Autodesk Inventor part; units mm, degrees
(part 2 of 3)
  line L905 (15.1918, 12.9829) -> (15.4759, 13.083)
  line L906 (15.4759, 13.083) -> (15.7953, 13.1808)
  line L907 (15.7953, 13.1808) -> (16.149, 13.2732)
  line L908 (16.149, 13.2732) -> (16.5404, 13.3581)
  line L909 (16.5404, 13.3581) -> (16.9661, 13.4319)
  line L910 (16.9661, 13.4319) -> (17.3813, 13.4867)
  arc A20 (18.1977, 12.3629) -> (17.3813, 13.4867) centre (0, 0) ccw
  line L911 (18.1977, 12.3629) -> (18.0173, 11.985)
  line L912 (18.0173, 11.985) -> (17.8155, 11.603)
  line L913 (17.8155, 11.603) -> (17.6139, 11.257)
  line L914 (17.6139, 11.257) -> (17.4167, 10.9491)
  line L915 (17.4167, 10.9491) -> (17.225, 10.6756)
  line L916 (17.225, 10.6756) -> (17.042, 10.4364)
  line L917 (17.042, 10.4364) -> (16.8707, 10.231)
  line L918 (16.8707, 10.231) -> (16.7119, 10.0559)
  line L919 (16.7119, 10.0559) -> (16.5707, 9.9128)
  line L920 (16.5707, 9.9128) -> (16.3443, 9.7094)
  line L921 (16.3443, 9.7094) -> (16.2048, 9.6033)
  line L922 (16.2048, 9.6033) -> (16.0637, 9.5056)
  line L923 (16.0637, 9.5056) -> (15.8979, 9.3692)
  line L924 (15.8979, 9.3692) -> (15.7712, 9.237)
  line L925 (15.7712, 9.237) -> (15.7224, 9.1734)
  line L926 (15.7224, 9.1734) -> (15.6831, 9.112)
  line L927 (15.6831, 9.112) -> (15.6531, 9.0532)
  line L928 (15.6531, 9.0532) -> (15.6325, 8.9973)
  line L929 (15.6325, 8.9973) -> (15.621, 8.9446)
  line L930 (15.621, 8.9446) -> (15.6184, 8.8956)
  line L931 (15.6184, 8.8956) -> (15.6247, 8.8505)
  line L932 (15.6247, 8.8505) -> (15.6447, 8.8003)
  line L933 (15.6447, 8.8003) -> (15.7975, 8.5231)
  line L934 (15.7975, 8.5231) -> (15.9936, 8.1491)
  line L935 (15.9936, 8.1491) -> (16.1809, 7.7707)
  line L936 (16.1809, 7.7707) -> (16.3153, 7.4841)
  line L937 (16.3153, 7.4841) -> (16.3442, 7.4385)
  line L938 (16.3442, 7.4385) -> (16.3769, 7.4069)
  line L939 (16.3769, 7.4069) -> (16.4181, 7.3801)
  line L940 (16.4181, 7.3801) -> (16.4675, 7.3585)
  line L941 (16.4675, 7.3585) -> (16.5249, 7.3423)
  line L942 (16.5249, 7.3423) -> (16.5901, 7.3319)
  line L943 (16.5901, 7.3319) -> (16.6629, 7.3277)
  line L944 (16.6629, 7.3277) -> (16.743, 7.3298)
  line L945 (16.743, 7.3298) -> (16.9244, 7.3546)
  line L946 (16.9244, 7.3546) -> (17.1322, 7.4085)
  line L947 (17.1322, 7.4085) -> (17.2942, 7.4653)
  line L948 (17.2942, 7.4653) -> (17.462, 7.5158)
  line L949 (17.462, 7.5158) -> (17.7596, 7.5794)
  line L950 (17.7596, 7.5794) -> (17.9584, 7.6095)
  line L951 (17.9584, 7.6095) -> (18.1934, 7.6351)
  line L952 (18.1934, 7.6351) -> (18.4602, 7.6529)
  line L953 (18.4602, 7.6529) -> (18.7613, 7.6604)
  line L954 (18.7613, 7.6604) -> (19.0953, 7.6547)
  line L955 (19.0953, 7.6547) -> (19.4602, 7.6332)
  line L956 (19.4602, 7.6332) -> (19.8587, 7.593)
  line L957 (19.8587, 7.593) -> (20.2864, 7.5317)
  line L958 (20.2864, 7.5317) -> (20.6982, 7.4555)
  arc A21 (21.1274, 6.1345) -> (20.6982, 7.4555) centre (0, 0) ccw
  line L959 (21.1274, 6.1345) -> (20.839, 5.8308)
  line L960 (20.839, 5.8308) -> (20.5291, 5.5298)
  line L961 (20.5291, 5.5298) -> (20.2304, 5.263)
  line L962 (20.2304, 5.263) -> (19.9477, 5.0311)
  line L963 (19.9477, 5.0311) -> (19.6809, 4.8302)
  line L964 (19.6809, 4.8302) -> (19.4329, 4.6593)
  line L965 (19.4329, 4.6593) -> (19.2065, 4.5169)
  line L966 (19.2065, 4.5169) -> (19.0014, 4.3995)
  line L967 (19.0014, 4.3995) -> (18.8229, 4.307)
  line L968 (18.8229, 4.307) -> (18.5448, 4.1835)
  line L969 (18.5448, 4.1835) -> (18.3792, 4.1257)
  line L970 (18.3792, 4.1257) -> (18.2149, 4.0764)
  line L971 (18.2149, 4.0764) -> (18.015, 3.9979)
  line L972 (18.015, 3.9979) -> (17.8537, 3.9113)
  line L973 (17.8537, 3.9113) -> (17.7876, 3.866)
  line L974 (17.7876, 3.866) -> (17.7313, 3.8197)
  line L975 (17.7313, 3.8197) -> (17.6846, 3.773)
  line L976 (17.6846, 3.773) -> (17.6477, 3.7262)
  line L977 (17.6477, 3.7262) -> (17.6205, 3.6797)
  line L978 (17.6205, 3.6797) -> (17.6029, 3.6338)
  line L979 (17.6029, 3.6338) -> (17.5949, 3.589)
  line L980 (17.5949, 3.589) -> (17.5985, 3.5351)
  line L981 (17.5985, 3.5351) -> (17.6581, 3.2242)
  line L982 (17.6581, 3.2242) -> (17.729, 2.808)
  line L983 (17.729, 2.808) -> (17.7902, 2.3902)
  line L984 (17.7902, 2.3902) -> (17.8295, 2.0761)
  line L985 (17.8295, 2.0761) -> (17.8429, 2.0238)
  line L986 (17.8429, 2.0238) -> (17.8643, 1.9836)
  line L987 (17.8643, 1.9836) -> (17.8951, 1.9454)
  line L988 (17.8951, 1.9454) -> (17.9354, 1.9096)
  line L989 (17.9354, 1.9096) -> (17.985, 1.8765)
  line L990 (17.985, 1.8765) -> (18.0438, 1.8465)
  line L991 (18.0438, 1.8465) -> (18.1117, 1.8199)
  line L992 (18.1117, 1.8199) -> (18.1886, 1.7972)
  line L993 (18.1886, 1.7972) -> (18.3687, 1.7647)
  line L994 (18.3687, 1.7647) -> (18.583, 1.7518)
  line L995 (18.583, 1.7518) -> (18.7546, 1.7557)
  line L996 (18.7546, 1.7557) -> (18.9299, 1.7519)
  line L997 (18.9299, 1.7519) -> (19.2325, 1.7204)
  line L998 (19.2325, 1.7204) -> (19.4309, 1.6876)
  line L999 (19.4309, 1.6876) -> (19.6623, 1.6393)
  line L1000 (19.6623, 1.6393) -> (19.9216, 1.5738)
  line L1001 (19.9216, 1.5738) -> (20.2103, 1.4879)
  line L1002 (20.2103, 1.4879) -> (20.5261, 1.3793)
  line L1003 (20.5261, 1.3793) -> (20.8666, 1.2461)
  line L1004 (20.8666, 1.2461) -> (21.2331, 1.0847)
  line L1005 (21.2331, 1.0847) -> (21.6209, 0.8942)
  line L1006 (21.6209, 0.8942) -> (21.989, 0.6945)
  arc A22 (21.989, -0.6945) -> (21.989, 0.6945) centre (0, 0) ccw
  line L1007 (21.989, -0.6945) -> (21.6209, -0.8942)
  line L1008 (21.6209, -0.8942) -> (21.2331, -1.0847)
  line L1009 (21.2331, -1.0847) -> (20.8666, -1.2461)
  line L1010 (20.8666, -1.2461) -> (20.5261, -1.3793)
  line L1011 (20.5261, -1.3793) -> (20.2103, -1.4879)
  line L1012 (20.2103, -1.4879) -> (19.9216, -1.5738)
  line L1013 (19.9216, -1.5738) -> (19.6623, -1.6393)
  line L1014 (19.6623, -1.6393) -> (19.4309, -1.6876)
  line L1015 (19.4309, -1.6876) -> (19.2325, -1.7204)
  line L1016 (19.2325, -1.7204) -> (18.9299, -1.7519)
  line L1017 (18.9299, -1.7519) -> (18.7546, -1.7557)
  line L1018 (18.7546, -1.7557) -> (18.583, -1.7518)
  line L1019 (18.583, -1.7518) -> (18.3687, -1.7647)
  line L1020 (18.3687, -1.7647) -> (18.1886, -1.7972)
  line L1021 (18.1886, -1.7972) -> (18.1117, -1.8199)
  line L1022 (18.1117, -1.8199) -> (18.0438, -1.8465)
  line L1023 (18.0438, -1.8465) -> (17.985, -1.8765)
  line L1024 (17.985, -1.8765) -> (17.9354, -1.9096)
  line L1025 (17.9354, -1.9096) -> (17.8951, -1.9454)
  line L1026 (17.8951, -1.9454) -> (17.8643, -1.9836)
  line L1027 (17.8643, -1.9836) -> (17.8429, -2.0238)
  line L1028 (17.8429, -2.0238) -> (17.8295, -2.0761)
  line L1029 (17.8295, -2.0761) -> (17.7902, -2.3902)
  line L1030 (17.7902, -2.3902) -> (17.729, -2.808)
  line L1031 (17.729, -2.808) -> (17.6581, -3.2242)
  line L1032 (17.6581, -3.2242) -> (17.5985, -3.5351)
  line L1033 (17.5985, -3.5351) -> (17.5949, -3.589)
  line L1034 (17.5949, -3.589) -> (17.6029, -3.6338)
  line L1035 (17.6029, -3.6338) -> (17.6205, -3.6797)
  line L1036 (17.6205, -3.6797) -> (17.6477, -3.7262)
  line L1037 (17.6477, -3.7262) -> (17.6846, -3.773)
  line L1038 (17.6846, -3.773) -> (17.7313, -3.8197)
  line L1039 (17.7313, -3.8197) -> (17.7876, -3.866)
  line L1040 (17.7876, -3.866) -> (17.8537, -3.9113)
  line L1041 (17.8537, -3.9113) -> (18.015, -3.9979)
  line L1042 (18.015, -3.9979) -> (18.2149, -4.0764)
  line L1043 (18.2149, -4.0764) -> (18.3792, -4.1257)
  line L1044 (18.3792, -4.1257) -> (18.5448, -4.1835)
  line L1045 (18.5448, -4.1835) -> (18.8229, -4.307)
  line L1046 (18.8229, -4.307) -> (19.0014, -4.3995)
  line L1047 (19.0014, -4.3995) -> (19.2065, -4.5169)
  line L1048 (19.2065, -4.5169) -> (19.4329, -4.6593)
  line L1049 (19.4329, -4.6593) -> (19.6809, -4.8302)
  line L1050 (19.6809, -4.8302) -> (19.9477, -5.0311)
  line L1051 (19.9477, -5.0311) -> (20.2304, -5.263)
  line L1052 (20.2304, -5.263) -> (20.5291, -5.5298)
  line L1053 (20.5291, -5.5298) -> (20.839, -5.8308)
  line L1054 (20.839, -5.8308) -> (21.1274, -6.1345)
  arc A23 (20.6982, -7.4555) -> (21.1274, -6.1345) centre (0, 0) ccw
  line L1055 (20.6982, -7.4555) -> (20.2864, -7.5317)
  line L1056 (20.2864, -7.5317) -> (19.8587, -7.593)
  line L1057 (19.8587, -7.593) -> (19.4602, -7.6332)
  line L1058 (19.4602, -7.6332) -> (19.0953, -7.6547)
  line L1059 (19.0953, -7.6547) -> (18.7613, -7.6604)
  line L1060 (18.7613, -7.6604) -> (18.4602, -7.6529)
  line L1061 (18.4602, -7.6529) -> (18.1934, -7.6351)
  line L1062 (18.1934, -7.6351) -> (17.9584, -7.6095)
  line L1063 (17.9584, -7.6095) -> (17.7596, -7.5794)
  line L1064 (17.7596, -7.5794) -> (17.462, -7.5158)
  line L1065 (17.462, -7.5158) -> (17.2942, -7.4653)
  line L1066 (17.2942, -7.4653) -> (17.1322, -7.4085)
  line L1067 (17.1322, -7.4085) -> (16.9244, -7.3546)
  line L1068 (16.9244, -7.3546) -> (16.743, -7.3298)
  line L1069 (16.743, -7.3298) -> (16.6629, -7.3277)
  line L1070 (16.6629, -7.3277) -> (16.5901, -7.3319)
  line L1071 (16.5901, -7.3319) -> (16.5249, -7.3423)
  line L1072 (16.5249, -7.3423) -> (16.4675, -7.3585)
  line L1073 (16.4675, -7.3585) -> (16.4181, -7.3801)
  line L1074 (16.4181, -7.3801) -> (16.3769, -7.4069)
  line L1075 (16.3769, -7.4069) -> (16.3442, -7.4385)
  line L1076 (16.3442, -7.4385) -> (16.3153, -7.4841)
  line L1077 (16.3153, -7.4841) -> (16.1809, -7.7707)
  line L1078 (16.1809, -7.7707) -> (15.9936, -8.1491)
  line L1079 (15.9936, -8.1491) -> (15.7975, -8.5231)
  line L1080 (15.7975, -8.5231) -> (15.6447, -8.8003)
  line L1081 (15.6447, -8.8003) -> (15.6247, -8.8505)
  line L1082 (15.6247, -8.8505) -> (15.6184, -8.8956)
  line L1083 (15.6184, -8.8956) -> (15.621, -8.9446)
  line L1084 (15.621, -8.9446) -> (15.6325, -8.9973)
  line L1085 (15.6325, -8.9973) -> (15.6531, -9.0532)
  line L1086 (15.6531, -9.0532) -> (15.6831, -9.112)
  line L1087 (15.6831, -9.112) -> (15.7224, -9.1734)
  line L1088 (15.7224, -9.1734) -> (15.7712, -9.237)
  line L1089 (15.7712, -9.237) -> (15.8979, -9.3692)
  line L1090 (15.8979, -9.3692) -> (16.0637, -9.5056)
  line L1091 (16.0637, -9.5056) -> (16.2048, -9.6033)
  line L1092 (16.2048, -9.6033) -> (16.3443, -9.7094)
  line L1093 (16.3443, -9.7094) -> (16.5707, -9.9128)
  line L1094 (16.5707, -9.9128) -> (16.7119, -10.0559)
  line L1095 (16.7119, -10.0559) -> (16.8707, -10.231)
  line L1096 (16.8707, -10.231) -> (17.042, -10.4364)
  line L1097 (17.042, -10.4364) -> (17.225, -10.6756)
  line L1098 (17.225, -10.6756) -> (17.4167, -10.9491)
  line L1099 (17.4167, -10.9491) -> (17.6139, -11.257)
  line L1100 (17.6139, -11.257) -> (17.8155, -11.603)
  line L1101 (17.8155, -11.603) -> (18.0173, -11.985)
  line L1102 (18.0173, -11.985) -> (18.1977, -12.3629)
  arc A24 (17.3813, -13.4867) -> (18.1977, -12.3629) centre (0, 0) ccw
  line L1103 (17.3813, -13.4867) -> (16.9661, -13.4319)
  line L1104 (16.9661, -13.4319) -> (16.5404, -13.3581)
  line L1105 (16.5404, -13.3581) -> (16.149, -13.2732)
  line L1106 (16.149, -13.2732) -> (15.7953, -13.1808)
  line L1107 (15.7953, -13.1808) -> (15.4759, -13.083)
  line L1108 (15.4759, -13.083) -> (15.1918, -12.9829)
  line L1109 (15.1918, -12.9829) -> (14.9436, -12.8835)
  line L1110 (14.9436, -12.8835) -> (14.728, -12.7865)
  line L1111 (14.728, -12.7865) -> (14.5482, -12.6964)
  line L1112 (14.5482, -12.6964) -> (14.2849, -12.544)
  line L1113 (14.2849, -12.544) -> (14.1408, -12.4441)
  line L1114 (14.1408, -12.4441) -> (14.0043, -12.3401)
  line L1115 (14.0043, -12.3401) -> (13.8234, -12.2245)
  line L1116 (13.8234, -12.2245) -> (13.6585, -12.1449)
  line L1117 (13.6585, -12.1449) -> (13.5829, -12.1181)
  line L1118 (13.5829, -12.1181) -> (13.5124, -12.0997)
  line L1119 (13.5124, -12.0997) -> (13.4472, -12.0894)
  line L1120 (13.4472, -12.0894) -> (13.3876, -12.0871)
  line L1121 (13.3876, -12.0871) -> (13.334, -12.0924)
  line L1122 (13.334, -12.0924) -> (13.2865, -12.1051)
  line L1123 (13.2865, -12.1051) -> (13.2456, -12.125)
  line L1124 (13.2456, -12.125) -> (13.2041, -12.1596)
  line L1125 (13.2041, -12.1596) -> (12.9876, -12.3906)
  line L1126 (12.9876, -12.3906) -> (12.6926, -12.6926)
  line L1127 (12.6926, -12.6926) -> (12.3906, -12.9876)
  line L1128 (12.3906, -12.9876) -> (12.1596, -13.2041)
  line L1129 (12.1596, -13.2041) -> (12.125, -13.2456)
  line L1130 (12.125, -13.2456) -> (12.1051, -13.2865)
  line L1131 (12.1051, -13.2865) -> (12.0924, -13.334)
  line L1132 (12.0924, -13.334) -> (12.0871, -13.3876)
  line L1133 (12.0871, -13.3876) -> (12.0894, -13.4472)
  line L1134 (12.0894, -13.4472) -> (12.0997, -13.5124)
  line L1135 (12.0997, -13.5124) -> (12.1181, -13.5829)
  line L1136 (12.1181, -13.5829) -> (12.1449, -13.6585)
  line L1137 (12.1449, -13.6585) -> (12.2245, -13.8234)
  line L1138 (12.2245, -13.8234) -> (12.3401, -14.0043)
  line L1139 (12.3401, -14.0043) -> (12.4441, -14.1408)
  line L1140 (12.4441, -14.1408) -> (12.544, -14.2849)
  line L1141 (12.544, -14.2849) -> (12.6964, -14.5482)
  line L1142 (12.6964, -14.5482) -> (12.7865, -14.728)
  line L1143 (12.7865, -14.728) -> (12.8835, -14.9436)
  line L1144 (12.8835, -14.9436) -> (12.9829, -15.1918)
  line L1145 (12.9829, -15.1918) -> (13.083, -15.4759)
  line L1146 (13.083, -15.4759) -> (13.1808, -15.7953)
  line L1147 (13.1808, -15.7953) -> (13.2732, -16.149)
  line L1148 (13.2732, -16.149) -> (13.3581, -16.5404)
  line L1149 (13.3581, -16.5404) -> (13.4319, -16.9661)
  line L1150 (13.4319, -16.9661) -> (13.4867, -17.3813)
  arc A25 (12.3629, -18.1977) -> (13.4867, -17.3813) centre (0, 0) ccw
  line L1151 (12.3629, -18.1977) -> (11.985, -18.0173)
  line L1152 (11.985, -18.0173) -> (11.603, -17.8155)
  line L1153 (11.603, -17.8155) -> (11.257, -17.6139)
  line L1154 (11.257, -17.6139) -> (10.9491, -17.4167)
  line L1155 (10.9491, -17.4167) -> (10.6756, -17.225)
  line L1156 (10.6756, -17.225) -> (10.4364, -17.042)
  line L1157 (10.4364, -17.042) -> (10.231, -16.8707)
  line L1158 (10.231, -16.8707) -> (10.0559, -16.7119)
  line L1159 (10.0559, -16.7119) -> (9.9128, -16.5707)
  line L1160 (9.9128, -16.5707) -> (9.7094, -16.3443)
  line L1161 (9.7094, -16.3443) -> (9.6033, -16.2048)
  line L1162 (9.6033, -16.2048) -> (9.5056, -16.0637)
  line L1163 (9.5056, -16.0637) -> (9.3692, -15.8979)
  line L1164 (9.3692, -15.8979) -> (9.237, -15.7712)
  line L1165 (9.237, -15.7712) -> (9.1734, -15.7224)
  line L1166 (9.1734, -15.7224) -> (9.112, -15.6831)
  line L1167 (9.112, -15.6831) -> (9.0532, -15.6531)
  line L1168 (9.0532, -15.6531) -> (8.9973, -15.6325)
  line L1169 (8.9973, -15.6325) -> (8.9446, -15.621)
  line L1170 (8.9446, -15.621) -> (8.8956, -15.6184)
  line L1171 (8.8956, -15.6184) -> (8.8505, -15.6247)
  line L1172 (8.8505, -15.6247) -> (8.8003, -15.6447)
  line L1173 (8.8003, -15.6447) -> (8.5231, -15.7975)
  line L1174 (8.5231, -15.7975) -> (8.1491, -15.9936)
  line L1175 (8.1491, -15.9936) -> (7.7707, -16.1809)
  line L1176 (7.7707, -16.1809) -> (7.4841, -16.3153)
  line L1177 (7.4841, -16.3153) -> (7.4385, -16.3442)
  line L1178 (7.4385, -16.3442) -> (7.4069, -16.3769)
  line L1179 (7.4069, -16.3769) -> (7.3801, -16.4181)
  line L1180 (7.3801, -16.4181) -> (7.3585, -16.4675)
  line L1181 (7.3585, -16.4675) -> (7.3423, -16.5249)
  line L1182 (7.3423, -16.5249) -> (7.3319, -16.5901)
  line L1183 (7.3319, -16.5901) -> (7.3277, -16.6629)
  line L1184 (7.3277, -16.6629) -> (7.3298, -16.743)
  line L1185 (7.3298, -16.743) -> (7.3546, -16.9244)
  line L1186 (7.3546, -16.9244) -> (7.4085, -17.1322)
  line L1187 (7.4085, -17.1322) -> (7.4653, -17.2942)
  line L1188 (7.4653, -17.2942) -> (7.5158, -17.462)
  line L1189 (7.5158, -17.462) -> (7.5794, -17.7596)
  line L1190 (7.5794, -17.7596) -> (7.6095, -17.9584)
  line L1191 (7.6095, -17.9584) -> (7.6351, -18.1934)
  line L1192 (7.6351, -18.1934) -> (7.6529, -18.4602)
  line L1193 (7.6529, -18.4602) -> (7.6604, -18.7613)
  line L1194 (7.6604, -18.7613) -> (7.6547, -19.0953)
  line L1195 (7.6547, -19.0953) -> (7.6332, -19.4602)
  line L1196 (7.6332, -19.4602) -> (7.593, -19.8587)
  line L1197 (7.593, -19.8587) -> (7.5317, -20.2864)
  line L1198 (7.5317, -20.2864) -> (7.4555, -20.6982)
  arc A26 (6.1345, -21.1274) -> (7.4555, -20.6982) centre (0, 0) ccw
  line L1199 (6.1345, -21.1274) -> (5.8308, -20.839)
  line L1200 (5.8308, -20.839) -> (5.5298, -20.5291)
  line L1201 (5.5298, -20.5291) -> (5.263, -20.2304)
  line L1202 (5.263, -20.2304) -> (5.0311, -19.9477)
  line L1203 (5.0311, -19.9477) -> (4.8302, -19.6809)
  line L1204 (4.8302, -19.6809) -> (4.6593, -19.4329)
  line L1205 (4.6593, -19.4329) -> (4.5169, -19.2065)
  line L1206 (4.5169, -19.2065) -> (4.3995, -19.0014)
  line L1207 (4.3995, -19.0014) -> (4.307, -18.8229)
  line L1208 (4.307, -18.8229) -> (4.1835, -18.5448)
  line L1209 (4.1835, -18.5448) -> (4.1257, -18.3792)
  line L1210 (4.1257, -18.3792) -> (4.0764, -18.2149)
  line L1211 (4.0764, -18.2149) -> (3.9979, -18.015)
  line L1212 (3.9979, -18.015) -> (3.9113, -17.8537)
  line L1213 (3.9113, -17.8537) -> (3.866, -17.7876)
  line L1214 (3.866, -17.7876) -> (3.8197, -17.7313)
  line L1215 (3.8197, -17.7313) -> (3.773, -17.6846)
  line L1216 (3.773, -17.6846) -> (3.7262, -17.6477)
  line L1217 (3.7262, -17.6477) -> (3.6797, -17.6205)
  line L1218 (3.6797, -17.6205) -> (3.6338, -17.6029)
  line L1219 (3.6338, -17.6029) -> (3.589, -17.5949)
  line L1220 (3.589, -17.5949) -> (3.5351, -17.5985)
  line L1221 (3.5351, -17.5985) -> (3.2242, -17.6581)
  line L1222 (3.2242, -17.6581) -> (2.808, -17.729)
  line L1223 (2.808, -17.729) -> (2.3902, -17.7902)
  line L1224 (2.3902, -17.7902) -> (2.0761, -17.8295)
  line L1225 (2.0761, -17.8295) -> (2.0238, -17.8429)
  line L1226 (2.0238, -17.8429) -> (1.9836, -17.8643)
  line L1227 (1.9836, -17.8643) -> (1.9454, -17.8951)
  line L1228 (1.9454, -17.8951) -> (1.9096, -17.9354)
  line L1229 (1.9096, -17.9354) -> (1.8765, -17.985)
  line L1230 (1.8765, -17.985) -> (1.8465, -18.0438)
  line L1231 (1.8465, -18.0438) -> (1.8199, -18.1117)
  line L1232 (1.8199, -18.1117) -> (1.7972, -18.1886)
  line L1233 (1.7972, -18.1886) -> (1.7647, -18.3687)
  line L1234 (1.7647, -18.3687) -> (1.7518, -18.583)
  line L1235 (1.7518, -18.583) -> (1.7557, -18.7546)
  line L1236 (1.7557, -18.7546) -> (1.7519, -18.9299)
  line L1237 (1.7519, -18.9299) -> (1.7204, -19.2325)
  line L1238 (1.7204, -19.2325) -> (1.6876, -19.4309)
  line L1239 (1.6876, -19.4309) -> (1.6393, -19.6623)
  line L1240 (1.6393, -19.6623) -> (1.5738, -19.9216)
  line L1241 (1.5738, -19.9216) -> (1.4879, -20.2103)
  line L1242 (1.4879, -20.2103) -> (1.3793, -20.5261)
  line L1243 (1.3793, -20.5261) -> (1.2461, -20.8666)
  line L1244 (1.2461, -20.8666) -> (1.0847, -21.2331)
  line L1245 (1.0847, -21.2331) -> (0.8942, -21.6209)
  line L1246 (0.8942, -21.6209) -> (0.6945, -21.989)
  arc A27 (-0.6945, -21.989) -> (0.6945, -21.989) centre (0, 0) ccw
  line L1247 (-0.6945, -21.989) -> (-0.8942, -21.6209)
  line L1248 (-0.8942, -21.6209) -> (-1.0847, -21.2331)
  line L1249 (-1.0847, -21.2331) -> (-1.2461, -20.8666)
  line L1250 (-1.2461, -20.8666) -> (-1.3793, -20.5261)
  line L1251 (-1.3793, -20.5261) -> (-1.4879, -20.2103)
  line L1252 (-1.4879, -20.2103) -> (-1.5738, -19.9216)
  line L1253 (-1.5738, -19.9216) -> (-1.6393, -19.6623)
  line L1254 (-1.6393, -19.6623) -> (-1.6876, -19.4309)
  line L1255 (-1.6876, -19.4309) -> (-1.7204, -19.2325)
  line L1256 (-1.7204, -19.2325) -> (-1.7519, -18.9299)
  line L1257 (-1.7519, -18.9299) -> (-1.7557, -18.7546)
  line L1258 (-1.7557, -18.7546) -> (-1.7518, -18.583)
  line L1259 (-1.7518, -18.583) -> (-1.7647, -18.3687)
  line L1260 (-1.7647, -18.3687) -> (-1.7972, -18.1886)
  line L1261 (-1.7972, -18.1886) -> (-1.8199, -18.1117)
  line L1262 (-1.8199, -18.1117) -> (-1.8465, -18.0438)
  line L1263 (-1.8465, -18.0438) -> (-1.8765, -17.985)
  line L1264 (-1.8765, -17.985) -> (-1.9096, -17.9354)
  line L1265 (-1.9096, -17.9354) -> (-1.9454, -17.8951)
  line L1266 (-1.9454, -17.8951) -> (-1.9836, -17.8643)
  line L1267 (-1.9836, -17.8643) -> (-2.0238, -17.8429)
  line L1268 (-2.0238, -17.8429) -> (-2.0761, -17.8295)
  line L1269 (-2.0761, -17.8295) -> (-2.3902, -17.7902)
  line L1270 (-2.3902, -17.7902) -> (-2.808, -17.729)
  line L1271 (-2.808, -17.729) -> (-3.2242, -17.6581)
  line L1272 (-3.2242, -17.6581) -> (-3.5351, -17.5985)
  line L1273 (-3.5351, -17.5985) -> (-3.589, -17.5949)
  line L1274 (-3.589, -17.5949) -> (-3.6338, -17.6029)
  line L1275 (-3.6338, -17.6029) -> (-3.6797, -17.6205)
  line L1276 (-3.6797, -17.6205) -> (-3.7262, -17.6477)
  line L1277 (-3.7262, -17.6477) -> (-3.773, -17.6846)
  line L1278 (-3.773, -17.6846) -> (-3.8197, -17.7313)
  line L1279 (-3.8197, -17.7313) -> (-3.866, -17.7876)
  line L1280 (-3.866, -17.7876) -> (-3.9113, -17.8537)
  line L1281 (-3.9113, -17.8537) -> (-3.9979, -18.015)
  line L1282 (-3.9979, -18.015) -> (-4.0764, -18.2149)
  line L1283 (-4.0764, -18.2149) -> (-4.1257, -18.3792)
  line L1284 (-4.1257, -18.3792) -> (-4.1835, -18.5448)
  line L1285 (-4.1835, -18.5448) -> (-4.307, -18.8229)
  line L1286 (-4.307, -18.8229) -> (-4.3995, -19.0014)
  line L1287 (-4.3995, -19.0014) -> (-4.5169, -19.2065)
  line L1288 (-4.5169, -19.2065) -> (-4.6593, -19.4329)
  line L1289 (-4.6593, -19.4329) -> (-4.8302, -19.6809)
  line L1290 (-4.8302, -19.6809) -> (-5.0311, -19.9477)
  line L1291 (-5.0311, -19.9477) -> (-5.263, -20.2304)
  line L1292 (-5.263, -20.2304) -> (-5.5298, -20.5291)
  line L1293 (-5.5298, -20.5291) -> (-5.8308, -20.839)
  line L1294 (-5.8308, -20.839) -> (-6.1345, -21.1274)
  arc A28 (-7.4555, -20.6982) -> (-6.1345, -21.1274) centre (0, 0) ccw
  line L1295 (-7.4555, -20.6982) -> (-7.5317, -20.2864)
  line L1296 (-7.5317, -20.2864) -> (-7.593, -19.8587)
  line L1297 (-7.593, -19.8587) -> (-7.6332, -19.4602)
  line L1298 (-7.6332, -19.4602) -> (-7.6547, -19.0953)
  line L1299 (-7.6547, -19.0953) -> (-7.6604, -18.7613)
  line L1300 (-7.6604, -18.7613) -> (-7.6529, -18.4602)
  line L1301 (-7.6529, -18.4602) -> (-7.6351, -18.1934)
  line L1302 (-7.6351, -18.1934) -> (-7.6095, -17.9584)
  line L1303 (-7.6095, -17.9584) -> (-7.5794, -17.7596)
  line L1304 (-7.5794, -17.7596) -> (-7.5158, -17.462)
  line L1305 (-7.5158, -17.462) -> (-7.4653, -17.2942)
  line L1306 (-7.4653, -17.2942) -> (-7.4085, -17.1322)
  line L1307 (-7.4085, -17.1322) -> (-7.3546, -16.9244)
  line L1308 (-7.3546, -16.9244) -> (-7.3298, -16.743)
  line L1309 (-7.3298, -16.743) -> (-7.3277, -16.6629)
  line L1310 (-7.3277, -16.6629) -> (-7.3319, -16.5901)
  line L1311 (-7.3319, -16.5901) -> (-7.3423, -16.5249)
  line L1312 (-7.3423, -16.5249) -> (-7.3585, -16.4675)
  line L1313 (-7.3585, -16.4675) -> (-7.3801, -16.4181)
  line L1314 (-7.3801, -16.4181) -> (-7.4069, -16.3769)
  line L1315 (-7.4069, -16.3769) -> (-7.4385, -16.3442)
  line L1316 (-7.4385, -16.3442) -> (-7.4841, -16.3153)
  line L1317 (-7.4841, -16.3153) -> (-7.7707, -16.1809)
  line L1318 (-7.7707, -16.1809) -> (-8.1491, -15.9936)
  line L1319 (-8.1491, -15.9936) -> (-8.5231, -15.7975)
  line L1320 (-8.5231, -15.7975) -> (-8.8003, -15.6447)
  line L1321 (-8.8003, -15.6447) -> (-8.8505, -15.6247)
  line L1322 (-8.8505, -15.6247) -> (-8.8956, -15.6184)
  line L1323 (-8.8956, -15.6184) -> (-8.9446, -15.621)
  line L1324 (-8.9446, -15.621) -> (-8.9973, -15.6325)
  line L1325 (-8.9973, -15.6325) -> (-9.0532, -15.6531)
  line L1326 (-9.0532, -15.6531) -> (-9.112, -15.6831)
  line L1327 (-9.112, -15.6831) -> (-9.1734, -15.7224)
  line L1328 (-9.1734, -15.7224) -> (-9.237, -15.7712)
  line L1329 (-9.237, -15.7712) -> (-9.3692, -15.8979)
  line L1330 (-9.3692, -15.8979) -> (-9.5056, -16.0637)
  line L1331 (-9.5056, -16.0637) -> (-9.6033, -16.2048)
  line L1332 (-9.6033, -16.2048) -> (-9.7094, -16.3443)
  line L1333 (-9.7094, -16.3443) -> (-9.9128, -16.5707)
  line L1334 (-9.9128, -16.5707) -> (-10.0559, -16.7119)
  line L1335 (-10.0559, -16.7119) -> (-10.231, -16.8707)
  line L1336 (-10.231, -16.8707) -> (-10.4364, -17.042)
  line L1337 (-10.4364, -17.042) -> (-10.6756, -17.225)
  line L1338 (-10.6756, -17.225) -> (-10.9491, -17.4167)
  line L1339 (-10.9491, -17.4167) -> (-11.257, -17.6139)
  line L1340 (-11.257, -17.6139) -> (-11.603, -17.8155)
  line L1341 (-11.603, -17.8155) -> (-11.985, -18.0173)
  line L1342 (-11.985, -18.0173) -> (-12.3629, -18.1977)
  arc A29 (-13.4867, -17.3813) -> (-12.3629, -18.1977) centre (0, 0) ccw
  line L1343 (-13.4867, -17.3813) -> (-13.4319, -16.9661)
  line L1344 (-13.4319, -16.9661) -> (-13.3581, -16.5404)
  line L1345 (-13.3581, -16.5404) -> (-13.2732, -16.149)
  line L1346 (-13.2732, -16.149) -> (-13.1808, -15.7953)
  line L1347 (-13.1808, -15.7953) -> (-13.083, -15.4759)
  line L1348 (-13.083, -15.4759) -> (-12.9829, -15.1918)
  line L1349 (-12.9829, -15.1918) -> (-12.8835, -14.9436)
  line L1350 (-12.8835, -14.9436) -> (-12.7865, -14.728)
  line L1351 (-12.7865, -14.728) -> (-12.6964, -14.5482)
  line L1352 (-12.6964, -14.5482) -> (-12.544, -14.2849)
  line L1353 (-12.544, -14.2849) -> (-12.4441, -14.1408)
  line L1354 (-12.4441, -14.1408) -> (-12.3401, -14.0043)
  line L1355 (-12.3401, -14.0043) -> (-12.2245, -13.8234)
  line L1356 (-12.2245, -13.8234) -> (-12.1449, -13.6585)
  line L1357 (-12.1449, -13.6585) -> (-12.1181, -13.5829)
  line L1358 (-12.1181, -13.5829) -> (-12.0997, -13.5124)
  line L1359 (-12.0997, -13.5124) -> (-12.0894, -13.4472)
  line L1360 (-12.0894, -13.4472) -> (-12.0871, -13.3876)
  line L1361 (-12.0871, -13.3876) -> (-12.0924, -13.334)
  line L1362 (-12.0924, -13.334) -> (-12.1051, -13.2865)
  line L1363 (-12.1051, -13.2865) -> (-12.125, -13.2456)
  line L1364 (-12.125, -13.2456) -> (-12.1596, -13.2041)
  line L1365 (-12.1596, -13.2041) -> (-12.3906, -12.9876)
  line L1366 (-12.3906, -12.9876) -> (-12.6926, -12.6926)
  line L1367 (-12.6926, -12.6926) -> (-12.9876, -12.3906)
  line L1368 (-12.9876, -12.3906) -> (-13.2041, -12.1596)
  line L1369 (-13.2041, -12.1596) -> (-13.2456, -12.125)
  line L1370 (-13.2456, -12.125) -> (-13.2865, -12.1051)
  line L1371 (-13.2865, -12.1051) -> (-13.334, -12.0924)
  line L1372 (-13.334, -12.0924) -> (-13.3876, -12.0871)
  line L1373 (-13.3876, -12.0871) -> (-13.4472, -12.0894)
  line L1374 (-13.4472, -12.0894) -> (-13.5124, -12.0997)
  line L1375 (-13.5124, -12.0997) -> (-13.5829, -12.1181)
  line L1376 (-13.5829, -12.1181) -> (-13.6585, -12.1449)
  line L1377 (-13.6585, -12.1449) -> (-13.8234, -12.2245)
  line L1378 (-13.8234, -12.2245) -> (-14.0043, -12.3401)
  line L1379 (-14.0043, -12.3401) -> (-14.1408, -12.4441)
  line L1380 (-14.1408, -12.4441) -> (-14.2849, -12.544)
  line L1381 (-14.2849, -12.544) -> (-14.5482, -12.6964)
  line L1382 (-14.5482, -12.6964) -> (-14.728, -12.7865)
  line L1383 (-14.728, -12.7865) -> (-14.9436, -12.8835)
  line L1384 (-14.9436, -12.8835) -> (-15.1918, -12.9829)
  line L1385 (-15.1918, -12.9829) -> (-15.4759, -13.083)
  line L1386 (-15.4759, -13.083) -> (-15.7953, -13.1808)
  line L1387 (-15.7953, -13.1808) -> (-16.149, -13.2732)
  line L1388 (-16.149, -13.2732) -> (-16.5404, -13.3581)
  line L1389 (-16.5404, -13.3581) -> (-16.9661, -13.4319)
  line L1390 (-16.9661, -13.4319) -> (-17.3813, -13.4867)
  arc A30 (-18.1977, -12.3629) -> (-17.3813, -13.4867) centre (0, 0) ccw
  line L1391 (-18.1977, -12.3629) -> (-18.0173, -11.985)
  line L1392 (-18.0173, -11.985) -> (-17.8155, -11.603)
  line L1393 (-17.8155, -11.603) -> (-17.6139, -11.257)
  line L1394 (-17.6139, -11.257) -> (-17.4167, -10.9491)
  line L1395 (-17.4167, -10.9491) -> (-17.225, -10.6756)
  line L1396 (-17.225, -10.6756) -> (-17.042, -10.4364)
  line L1397 (-17.042, -10.4364) -> (-16.8707, -10.231)
  line L1398 (-16.8707, -10.231) -> (-16.7119, -10.0559)
  line L1399 (-16.7119, -10.0559) -> (-16.5707, -9.9128)
  line L1400 (-16.5707, -9.9128) -> (-16.3443, -9.7094)
  line L1401 (-16.3443, -9.7094) -> (-16.2048, -9.6033)
  line L1402 (-16.2048, -9.6033) -> (-16.0637, -9.5056)
  line L1403 (-16.0637, -9.5056) -> (-15.8979, -9.3692)
  line L1404 (-15.8979, -9.3692) -> (-15.7712, -9.237)
  line L1405 (-15.7712, -9.237) -> (-15.7224, -9.1734)
  line L1406 (-15.7224, -9.1734) -> (-15.6831, -9.112)
  line L1407 (-15.6831, -9.112) -> (-15.6531, -9.0532)
  line L1408 (-15.6531, -9.0532) -> (-15.6325, -8.9973)
  line L1409 (-15.6325, -8.9973) -> (-15.621, -8.9446)
  line L1410 (-15.621, -8.9446) -> (-15.6184, -8.8956)
  line L1411 (-15.6184, -8.8956) -> (-15.6247, -8.8505)
  line L1412 (-15.6247, -8.8505) -> (-15.6447, -8.8003)
  line L1413 (-15.6447, -8.8003) -> (-15.7975, -8.5231)
  line L1414 (-15.7975, -8.5231) -> (-15.9936, -8.1491)
  line L1415 (-15.9936, -8.1491) -> (-16.1809, -7.7707)
  line L1416 (-16.1809, -7.7707) -> (-16.3153, -7.4841)
  line L1417 (-16.3153, -7.4841) -> (-16.3442, -7.4385)
  line L1418 (-16.3442, -7.4385) -> (-16.3769, -7.4069)
  line L1419 (-16.3769, -7.4069) -> (-16.4181, -7.3801)
  line L1420 (-16.4181, -7.3801) -> (-16.4675, -7.3585)
  line L1421 (-16.4675, -7.3585) -> (-16.5249, -7.3423)
  line L1422 (-16.5249, -7.3423) -> (-16.5901, -7.3319)
  line L1423 (-16.5901, -7.3319) -> (-16.6629, -7.3277)
  line L1424 (-16.6629, -7.3277) -> (-16.743, -7.3298)
  line L1425 (-16.743, -7.3298) -> (-16.9244, -7.3546)
  line L1426 (-16.9244, -7.3546) -> (-17.1322, -7.4085)
  line L1427 (-17.1322, -7.4085) -> (-17.2942, -7.4653)
  line L1428 (-17.2942, -7.4653) -> (-17.462, -7.5158)
  line L1429 (-17.462, -7.5158) -> (-17.7596, -7.5794)
  line L1430 (-17.7596, -7.5794) -> (-17.9584, -7.6095)
  line L1431 (-17.9584, -7.6095) -> (-18.1934, -7.6351)
  line L1432 (-18.1934, -7.6351) -> (-18.4602, -7.6529)
  line L1433 (-18.4602, -7.6529) -> (-18.7613, -7.6604)
  line L1434 (-18.7613, -7.6604) -> (-19.0953, -7.6547)
  line L1435 (-19.0953, -7.6547) -> (-19.4602, -7.6332)
  line L1436 (-19.4602, -7.6332) -> (-19.8587, -7.593)
  line L1437 (-19.8587, -7.593) -> (-20.2864, -7.5317)
  line L1438 (-20.2864, -7.5317) -> (-20.6982, -7.4555)
  arc A31 (-21.1274, -6.1345) -> (-20.6982, -7.4555) centre (0, 0) ccw
  line L1439 (-21.1274, -6.1345) -> (-20.839, -5.8308)
  line L1440 (-20.839, -5.8308) -> (-20.5291, -5.5298)
  line L1441 (-20.5291, -5.5298) -> (-20.2304, -5.263)
  line L1442 (-20.2304, -5.263) -> (-19.9477, -5.0311)
  line L1443 (-19.9477, -5.0311) -> (-19.6809, -4.8302)
  line L1444 (-19.6809, -4.8302) -> (-19.4329, -4.6593)
  line L1445 (-19.4329, -4.6593) -> (-19.2065, -4.5169)
  line L1446 (-19.2065, -4.5169) -> (-19.0014, -4.3995)
  line L1447 (-19.0014, -4.3995) -> (-18.8229, -4.307)
  line L1448 (-18.8229, -4.307) -> (-18.5448, -4.1835)
  line L1449 (-18.5448, -4.1835) -> (-18.3792, -4.1257)
  line L1450 (-18.3792, -4.1257) -> (-18.2149, -4.0764)
  line L1451 (-18.2149, -4.0764) -> (-18.015, -3.9979)
  line L1452 (-18.015, -3.9979) -> (-17.8537, -3.9113)
  line L1453 (-17.8537, -3.9113) -> (-17.7876, -3.866)
  line L1454 (-17.7876, -3.866) -> (-17.7313, -3.8197)
  line L1455 (-17.7313, -3.8197) -> (-17.6846, -3.773)
  line L1456 (-17.6846, -3.773) -> (-17.6477, -3.7262)
  line L1457 (-17.6477, -3.7262) -> (-17.6205, -3.6797)
  line L1458 (-17.6205, -3.6797) -> (-17.6029, -3.6338)
  line L1459 (-17.6029, -3.6338) -> (-17.5949, -3.589)
  line L1460 (-17.5949, -3.589) -> (-17.5985, -3.5351)
  line L1461 (-17.5985, -3.5351) -> (-17.6581, -3.2242)
  line L1462 (-17.6581, -3.2242) -> (-17.729, -2.808)
  line L1463 (-17.729, -2.808) -> (-17.7902, -2.3902)
  line L1464 (-17.7902, -2.3902) -> (-17.8295, -2.0761)
  line L1465 (-17.8295, -2.0761) -> (-17.8429, -2.0238)
  line L1466 (-17.8429, -2.0238) -> (-17.8643, -1.9836)
  line L1467 (-17.8643, -1.9836) -> (-17.8951, -1.9454)
  line L1468 (-17.8951, -1.9454) -> (-17.9354, -1.9096)
  line L1469 (-17.9354, -1.9096) -> (-17.985, -1.8765)
  line L1470 (-17.985, -1.8765) -> (-18.0438, -1.8465)
  line L1471 (-18.0438, -1.8465) -> (-18.1117, -1.8199)
  line L1472 (-18.1117, -1.8199) -> (-18.1886, -1.7972)
  line L1473 (-18.1886, -1.7972) -> (-18.3687, -1.7647)
  line L1474 (-18.3687, -1.7647) -> (-18.583, -1.7518)
  line L1475 (-18.583, -1.7518) -> (-18.7546, -1.7557)
  line L1476 (-18.7546, -1.7557) -> (-18.9299, -1.7519)
  line L1477 (-18.9299, -1.7519) -> (-19.2325, -1.7204)
  line L1478 (-19.2325, -1.7204) -> (-19.4309, -1.6876)
  line L1479 (-19.4309, -1.6876) -> (-19.6623, -1.6393)
  line L1480 (-19.6623, -1.6393) -> (-19.9216, -1.5738)
  line L1481 (-19.9216, -1.5738) -> (-20.2103, -1.4879)
  line L1482 (-20.2103, -1.4879) -> (-20.5261, -1.3793)
  line L1483 (-20.5261, -1.3793) -> (-20.8666, -1.2461)
  line L1484 (-20.8666, -1.2461) -> (-21.2331, -1.0847)
  line L1485 (-21.2331, -1.0847) -> (-21.6209, -0.8942)
  line L1486 (-21.6209, -0.8942) -> (-21.989, -0.6945)
  arc A32 (-21.989, 0.6945) -> (-21.989, -0.6945) centre (0, 0) ccw
  line L1487 (-21.989, 0.6945) -> (-21.6209, 0.8942)
  line L1488 (-21.6209, 0.8942) -> (-21.2331, 1.0847)
  line L1489 (-21.2331, 1.0847) -> (-20.8666, 1.2461)
  line L1490 (-20.8666, 1.2461) -> (-20.5261, 1.3793)
  line L1491 (-20.5261, 1.3793) -> (-20.2103, 1.4879)
  line L1492 (-20.2103, 1.4879) -> (-19.9216, 1.5738)
  line L1493 (-19.9216, 1.5738) -> (-19.6623, 1.6393)
  line L1494 (-19.6623, 1.6393) -> (-19.4309, 1.6876)
  line L1495 (-19.4309, 1.6876) -> (-19.2325, 1.7204)
  line L1496 (-19.2325, 1.7204) -> (-18.9299, 1.7519)
  line L1497 (-18.9299, 1.7519) -> (-18.7546, 1.7557)
  line L1498 (-18.7546, 1.7557) -> (-18.583, 1.7518)
  line L1499 (-18.583, 1.7518) -> (-18.3687, 1.7647)
  line L1500 (-18.3687, 1.7647) -> (-18.1886, 1.7972)
  line L1501 (-18.1886, 1.7972) -> (-18.1117, 1.8199)
  line L1502 (-18.1117, 1.8199) -> (-18.0438, 1.8465)
  line L1503 (-18.0438, 1.8465) -> (-17.985, 1.8765)
  line L1504 (-17.985, 1.8765) -> (-17.9354, 1.9096)
  line L1505 (-17.9354, 1.9096) -> (-17.8951, 1.9454)
  line L1506 (-17.8951, 1.9454) -> (-17.8643, 1.9836)
  line L1507 (-17.8643, 1.9836) -> (-17.8429, 2.0238)
  line L1508 (-17.8429, 2.0238) -> (-17.8295, 2.0761)
  line L1509 (-17.8295, 2.0761) -> (-17.7902, 2.3902)
  line L1510 (-17.7902, 2.3902) -> (-17.729, 2.808)
  line L1511 (-17.729, 2.808) -> (-17.6581, 3.2242)
  line L1512 (-17.6581, 3.2242) -> (-17.5985, 3.5351)
  line L1513 (-17.5985, 3.5351) -> (-17.5949, 3.589)
  line L1514 (-17.5949, 3.589) -> (-17.6029, 3.6338)
  line L1515 (-17.6029, 3.6338) -> (-17.6205, 3.6797)
  line L1516 (-17.6205, 3.6797) -> (-17.6477, 3.7262)
  line L1517 (-17.6477, 3.7262) -> (-17.6846, 3.773)
  line L1518 (-17.6846, 3.773) -> (-17.7313, 3.8197)
  line L1519 (-17.7313, 3.8197) -> (-17.7876, 3.866)
  line L1520 (-17.7876, 3.866) -> (-17.8537, 3.9113)
  line L1521 (-17.8537, 3.9113) -> (-18.015, 3.9979)
  line L1522 (-18.015, 3.9979) -> (-18.2149, 4.0764)
  line L1523 (-18.2149, 4.0764) -> (-18.3792, 4.1257)
  line L1524 (-18.3792, 4.1257) -> (-18.5448, 4.1835)
  line L1525 (-18.5448, 4.1835) -> (-18.8229, 4.307)
  line L1526 (-18.8229, 4.307) -> (-19.0014, 4.3995)
  line L1527 (-19.0014, 4.3995) -> (-19.2065, 4.5169)
  line L1528 (-19.2065, 4.5169) -> (-19.4329, 4.6593)
  line L1529 (-19.4329, 4.6593) -> (-19.6809, 4.8302)
  line L1530 (-19.6809, 4.8302) -> (-19.9477, 5.0311)
  line L1531 (-19.9477, 5.0311) -> (-20.2304, 5.263)
  line L1532 (-20.2304, 5.263) -> (-20.5291, 5.5298)
  line L1533 (-20.5291, 5.5298) -> (-20.839, 5.8308)
  line L1534 (-20.839, 5.8308) -> (-21.1274, 6.1345)
  arc A33 (-20.6982, 7.4555) -> (-21.1274, 6.1345) centre (0, 0) ccw
  line L1535 (-20.6982, 7.4555) -> (-20.2864, 7.5317)
  line L1536 (-20.2864, 7.5317) -> (-19.8587, 7.593)
  line L1537 (-19.8587, 7.593) -> (-19.4602, 7.6332)
  line L1538 (-19.4602, 7.6332) -> (-19.0953, 7.6547)
  line L1539 (-19.0953, 7.6547) -> (-18.7613, 7.6604)
  line L1540 (-18.7613, 7.6604) -> (-18.4602, 7.6529)
  line L1541 (-18.4602, 7.6529) -> (-18.1934, 7.6351)
  line L1542 (-18.1934, 7.6351) -> (-17.9584, 7.6095)
  line L1543 (-17.9584, 7.6095) -> (-17.7596, 7.5794)
  line L1544 (-17.7596, 7.5794) -> (-17.462, 7.5158)
  line L1545 (-17.462, 7.5158) -> (-17.2942, 7.4653)
  line L1546 (-17.2942, 7.4653) -> (-17.1322, 7.4085)
  line L1547 (-17.1322, 7.4085) -> (-16.9244, 7.3546)
  line L1548 (-16.9244, 7.3546) -> (-16.743, 7.3298)
  line L1549 (-16.743, 7.3298) -> (-16.6629, 7.3277)
  line L1550 (-16.6629, 7.3277) -> (-16.5901, 7.3319)
  line L1551 (-16.5901, 7.3319) -> (-16.5249, 7.3423)
  line L1552 (-16.5249, 7.3423) -> (-16.4675, 7.3585)
  line L1553 (-16.4675, 7.3585) -> (-16.4181, 7.3801)
  line L1554 (-16.4181, 7.3801) -> (-16.3769, 7.4069)
  line L1555 (-16.3769, 7.4069) -> (-16.3442, 7.4385)
  line L1556 (-16.3442, 7.4385) -> (-16.3153, 7.4841)
  line L1557 (-16.3153, 7.4841) -> (-16.1809, 7.7707)
  line L1558 (-16.1809, 7.7707) -> (-15.9936, 8.1491)
  line L1559 (-15.9936, 8.1491) -> (-15.7975, 8.5231)
  line L1560 (-15.7975, 8.5231) -> (-15.6447, 8.8003)
  line L1561 (-15.6447, 8.8003) -> (-15.6247, 8.8505)
  line L1562 (-15.6247, 8.8505) -> (-15.6184, 8.8956)
  line L1563 (-15.6184, 8.8956) -> (-15.621, 8.9446)
  line L1564 (-15.621, 8.9446) -> (-15.6325, 8.9973)
  line L1565 (-15.6325, 8.9973) -> (-15.6531, 9.0532)
  line L1566 (-15.6531, 9.0532) -> (-15.6831, 9.112)
  line L1567 (-15.6831, 9.112) -> (-15.7224, 9.1734)
  line L1568 (-15.7224, 9.1734) -> (-15.7712, 9.237)
  line L1569 (-15.7712, 9.237) -> (-15.8979, 9.3692)
  line L1570 (-15.8979, 9.3692) -> (-16.0637, 9.5056)
  line L1571 (-16.0637, 9.5056) -> (-16.2048, 9.6033)
  line L1572 (-16.2048, 9.6033) -> (-16.3443, 9.7094)
  line L1573 (-16.3443, 9.7094) -> (-16.5707, 9.9128)
  line L1574 (-16.5707, 9.9128) -> (-16.7119, 10.0559)
  line L1575 (-16.7119, 10.0559) -> (-16.8707, 10.231)
  line L1576 (-16.8707, 10.231) -> (-17.042, 10.4364)
  line L1577 (-17.042, 10.4364) -> (-17.225, 10.6756)
  line L1578 (-17.225, 10.6756) -> (-17.4167, 10.9491)
  line L1579 (-17.4167, 10.9491) -> (-17.6139, 11.257)
  line L1580 (-17.6139, 11.257) -> (-17.8155, 11.603)
  line L1581 (-17.8155, 11.603) -> (-18.0173, 11.985)
  line L1582 (-18.0173, 11.985) -> (-18.1977, 12.3629)
  arc A34 (-17.3813, 13.4867) -> (-18.1977, 12.3629) centre (0, 0) ccw
  line L1583 (-17.3813, 13.4867) -> (-16.9661, 13.4319)
  line L1584 (-16.9661, 13.4319) -> (-16.5404, 13.3581)
  line L1585 (-16.5404, 13.3581) -> (-16.149, 13.2732)
  line L1586 (-16.149, 13.2732) -> (-15.7953, 13.1808)
  line L1587 (-15.7953, 13.1808) -> (-15.4759, 13.083)
  line L1588 (-15.4759, 13.083) -> (-15.1918, 12.9829)
  line L1589 (-15.1918, 12.9829) -> (-14.9436, 12.8835)
  line L1590 (-14.9436, 12.8835) -> (-14.728, 12.7865)
  line L1591 (-14.728, 12.7865) -> (-14.5482, 12.6964)
  line L1592 (-14.5482, 12.6964) -> (-14.2849, 12.544)
  line L1593 (-14.2849, 12.544) -> (-14.1408, 12.4441)
  line L1594 (-14.1408, 12.4441) -> (-14.0043, 12.3401)
  line L1595 (-14.0043, 12.3401) -> (-13.8234, 12.2245)
  line L1596 (-13.8234, 12.2245) -> (-13.6585, 12.1449)
  line L1597 (-13.6585, 12.1449) -> (-13.5829, 12.1181)
  line L1598 (-13.5829, 12.1181) -> (-13.5124, 12.0997)
  line L1599 (-13.5124, 12.0997) -> (-13.4472, 12.0894)
  line L1600 (-13.4472, 12.0894) -> (-13.3876, 12.0871)
  line L1601 (-13.3876, 12.0871) -> (-13.334, 12.0924)
  line L1602 (-13.334, 12.0924) -> (-13.2865, 12.1051)
  line L1603 (-13.2865, 12.1051) -> (-13.2456, 12.125)
  line L1604 (-13.2456, 12.125) -> (-13.2041, 12.1596)
  line L1605 (-13.2041, 12.1596) -> (-12.9876, 12.3906)
  line L1606 (-12.9876, 12.3906) -> (-12.6926, 12.6926)
  line L1607 (-12.6926, 12.6926) -> (-12.3906, 12.9876)
  line L1608 (-12.3906, 12.9876) -> (-12.1596, 13.2041)
  line L1609 (-12.1596, 13.2041) -> (-12.125, 13.2456)
  line L1610 (-12.125, 13.2456) -> (-12.1051, 13.2865)
  line L1611 (-12.1051, 13.2865) -> (-12.0924, 13.334)
  line L1612 (-12.0924, 13.334) -> (-12.0871, 13.3876)
  line L1613 (-12.0871, 13.3876) -> (-12.0894, 13.4472)
  line L1614 (-12.0894, 13.4472) -> (-12.0997, 13.5124)
  line L1615 (-12.0997, 13.5124) -> (-12.1181, 13.5829)
  line L1616 (-12.1181, 13.5829) -> (-12.1449, 13.6585)
  line L1617 (-12.1449, 13.6585) -> (-12.2245, 13.8234)
  line L1618 (-12.2245, 13.8234) -> (-12.3401, 14.0043)
  line L1619 (-12.3401, 14.0043) -> (-12.4441, 14.1408)
  line L1620 (-12.4441, 14.1408) -> (-12.544, 14.2849)
  line L1621 (-12.544, 14.2849) -> (-12.6964, 14.5482)
  line L1622 (-12.6964, 14.5482) -> (-12.7865, 14.728)
  line L1623 (-12.7865, 14.728) -> (-12.8835, 14.9436)
  line L1624 (-12.8835, 14.9436) -> (-12.9829, 15.1918)
  line L1625 (-12.9829, 15.1918) -> (-13.083, 15.4759)
  line L1626 (-13.083, 15.4759) -> (-13.1808, 15.7953)
  line L1627 (-13.1808, 15.7953) -> (-13.2732, 16.149)
  line L1628 (-13.2732, 16.149) -> (-13.3581, 16.5404)
  line L1629 (-13.3581, 16.5404) -> (-13.4319, 16.9661)
  line L1630 (-13.4319, 16.9661) -> (-13.4867, 17.3813)
  arc A35 (-12.3629, 18.1977) -> (-13.4867, 17.3813) centre (0, 0) ccw
  line L1631 (-12.3629, 18.1977) -> (-11.985, 18.0173)
  line L1632 (-11.985, 18.0173) -> (-11.603, 17.8155)
  line L1633 (-11.603, 17.8155) -> (-11.257, 17.6139)
  line L1634 (-11.257, 17.6139) -> (-10.9491, 17.4167)
  line L1635 (-10.9491, 17.4167) -> (-10.6756, 17.225)
  line L1636 (-10.6756, 17.225) -> (-10.4364, 17.042)
  line L1637 (-10.4364, 17.042) -> (-10.231, 16.8707)
  line L1638 (-10.231, 16.8707) -> (-10.0559, 16.7119)
  line L1639 (-10.0559, 16.7119) -> (-9.9128, 16.5707)
  line L1640 (-9.9128, 16.5707) -> (-9.7094, 16.3443)
  line L1641 (-9.7094, 16.3443) -> (-9.6033, 16.2048)
  line L1642 (-9.6033, 16.2048) -> (-9.5056, 16.0637)
  line L1643 (-9.5056, 16.0637) -> (-9.3692, 15.8979)
  line L1644 (-9.3692, 15.8979) -> (-9.237, 15.7712)
  line L1645 (-9.237, 15.7712) -> (-9.1734, 15.7224)
  line L1646 (-9.1734, 15.7224) -> (-9.112, 15.6831)
  line L1647 (-9.112, 15.6831) -> (-9.0532, 15.6531)
  line L1648 (-9.0532, 15.6531) -> (-8.9973, 15.6325)
  line L1649 (-8.9973, 15.6325) -> (-8.9446, 15.621)
  line L1650 (-8.9446, 15.621) -> (-8.8956, 15.6184)
  line L1651 (-8.8956, 15.6184) -> (-8.8505, 15.6247)
  line L1652 (-8.8505, 15.6247) -> (-8.8003, 15.6447)
  line L1653 (-8.8003, 15.6447) -> (-8.5231, 15.7975)
  line L1654 (-8.5231, 15.7975) -> (-8.1491, 15.9936)
  line L1655 (-8.1491, 15.9936) -> (-7.7707, 16.1809)
  line L1656 (-7.7707, 16.1809) -> (-7.4841, 16.3153)
  line L1657 (-7.4841, 16.3153) -> (-7.4385, 16.3442)
  line L1658 (-7.4385, 16.3442) -> (-7.4069, 16.3769)
  line L1659 (-7.4069, 16.3769) -> (-7.3801, 16.4181)
  line L1660 (-7.3801, 16.4181) -> (-7.3585, 16.4675)
  line L1661 (-7.3585, 16.4675) -> (-7.3423, 16.5249)
  line L1662 (-7.3423, 16.5249) -> (-7.3319, 16.5901)
  line L1663 (-7.3319, 16.5901) -> (-7.3277, 16.6629)
  line L1664 (-7.3277, 16.6629) -> (-7.3298, 16.743)
  line L1665 (-7.3298, 16.743) -> (-7.3546, 16.9244)
  line L1666 (-7.3546, 16.9244) -> (-7.4085, 17.1322)
  line L1667 (-7.4085, 17.1322) -> (-7.4653, 17.2942)
  line L1668 (-7.4653, 17.2942) -> (-7.5158, 17.462)
  line L1669 (-7.5158, 17.462) -> (-7.5794, 17.7596)
  line L1670 (-7.5794, 17.7596) -> (-7.6095, 17.9584)
  line L1671 (-7.6095, 17.9584) -> (-7.6351, 18.1934)
  line L1672 (-7.6351, 18.1934) -> (-7.6529, 18.4602)
  line L1673 (-7.6529, 18.4602) -> (-7.6604, 18.7613)
  line L1674 (-7.6604, 18.7613) -> (-7.6547, 19.0953)
  line L1675 (-7.6547, 19.0953) -> (-7.6332, 19.4602)
  line L1676 (-7.6332, 19.4602) -> (-7.593, 19.8587)
  line L1677 (-7.593, 19.8587) -> (-7.5317, 20.2864)
  line L1678 (-7.5317, 20.2864) -> (-7.4555, 20.6982)
  arc A36 (-6.1345, 21.1274) -> (-7.4555, 20.6982) centre (0, 0) ccw
  line L1679 (-6.1345, 21.1274) -> (-5.8308, 20.839)
  line L1680 (-5.8308, 20.839) -> (-5.5298, 20.5291)
  line L1681 (-5.5298, 20.5291) -> (-5.263, 20.2304)
  line L1682 (-5.263, 20.2304) -> (-5.0311, 19.9477)
  line L1683 (-5.0311, 19.9477) -> (-4.8302, 19.6809)
  line L1684 (-4.8302, 19.6809) -> (-4.6593, 19.4329)
  line L1685 (-4.6593, 19.4329) -> (-4.5169, 19.2065)
  line L1686 (-4.5169, 19.2065) -> (-4.3995, 19.0014)
  line L1687 (-4.3995, 19.0014) -> (-4.307, 18.8229)
  line L1688 (-4.307, 18.8229) -> (-4.1835, 18.5448)
  line L1689 (-4.1835, 18.5448) -> (-4.1257, 18.3792)
  line L1690 (-4.1257, 18.3792) -> (-4.0764, 18.2149)
  line L1691 (-4.0764, 18.2149) -> (-3.9979, 18.015)
  line L1692 (-3.9979, 18.015) -> (-3.9113, 17.8537)
  line L1693 (-3.9113, 17.8537) -> (-3.866, 17.7876)
  line L1694 (-3.866, 17.7876) -> (-3.8197, 17.7313)
  line L1695 (-3.8197, 17.7313) -> (-3.773, 17.6846)
  line L1696 (-3.773, 17.6846) -> (-3.7262, 17.6477)
  line L1697 (-3.7262, 17.6477) -> (-3.6797, 17.6205)
  line L1698 (-3.6797, 17.6205) -> (-3.6338, 17.6029)
  line L1699 (-3.6338, 17.6029) -> (-3.589, 17.5949)
  line L1700 (-3.589, 17.5949) -> (-3.5351, 17.5985)
  line L1701 (-3.5351, 17.5985) -> (-3.2242, 17.6581)
  line L1702 (-3.2242, 17.6581) -> (-2.808, 17.729)
  line L1703 (-2.808, 17.729) -> (-2.3902, 17.7902)
  line L1704 (-2.3902, 17.7902) -> (-2.0761, 17.8295)
  line L1705 (-2.0761, 17.8295) -> (-2.0238, 17.8429)
  line L1706 (-2.0238, 17.8429) -> (-1.9836, 17.8643)
  line L1707 (-1.9836, 17.8643) -> (-1.9454, 17.8951)
  line L1708 (-1.9454, 17.8951) -> (-1.9096, 17.9354)
  line L1709 (-1.9096, 17.9354) -> (-1.8765, 17.985)
  line L1710 (-1.8765, 17.985) -> (-1.8465, 18.0438)
  line L1711 (-1.8465, 18.0438) -> (-1.8199, 18.1117)
  line L1712 (-1.8199, 18.1117) -> (-1.7972, 18.1886)
  line L1713 (-1.7972, 18.1886) -> (-1.7647, 18.3687)
  line L1714 (-1.7647, 18.3687) -> (-1.7518, 18.583)
  line L1715 (-1.7518, 18.583) -> (-1.7557, 18.7546)
  line L1716 (-1.7557, 18.7546) -> (-1.7519, 18.9299)
  line L1717 (-1.7519, 18.9299) -> (-1.7204, 19.2325)
  line L1718 (-1.7204, 19.2325) -> (-1.6876, 19.4309)
  line L1719 (-1.6876, 19.4309) -> (-1.6393, 19.6623)
  line L1720 (-1.6393, 19.6623) -> (-1.5738, 19.9216)
  line L1721 (-1.5738, 19.9216) -> (-1.4879, 20.2103)
  line L1722 (-1.4879, 20.2103) -> (-1.3793, 20.5261)
  line L1723 (-1.3793, 20.5261) -> (-1.2461, 20.8666)
  line L1724 (-1.2461, 20.8666) -> (-1.0847, 21.2331)
  line L1725 (-1.0847, 21.2331) -> (-0.8942, 21.6209)
  line L1726 (-0.8942, 21.6209) -> (-0.6945, 21.989)
  arc A37 (0.6945, 21.989) -> (-0.6945, 21.989) centre (0, 0) ccw
  line L1727 (0.6945, 21.989) -> (0.8942, 21.6209)
  line L1728 (0.8942, 21.6209) -> (1.0847, 21.2331)
  line L1729 (1.0847, 21.2331) -> (1.2461, 20.8666)
  line L1730 (1.2461, 20.8666) -> (1.3793, 20.5261)
  line L1731 (1.3793, 20.5261) -> (1.4879, 20.2103)
  line L1732 (1.4879, 20.2103) -> (1.5738, 19.9216)
  line L1733 (1.5738, 19.9216) -> (1.6393, 19.6623)
  line L1734 (1.6393, 19.6623) -> (1.6876, 19.4309)
  line L1735 (1.6876, 19.4309) -> (1.7204, 19.2325)
  line L1736 (1.7204, 19.2325) -> (1.7519, 18.9299)
  line L1737 (1.7519, 18.9299) -> (1.7557, 18.7546)
  line L1738 (1.7557, 18.7546) -> (1.7518, 18.583)
  line L1739 (1.7518, 18.583) -> (1.7647, 18.3687)
  line L1740 (1.7647, 18.3687) -> (1.7972, 18.1886)
  line L1741 (1.7972, 18.1886) -> (1.8199, 18.1117)
  line L1742 (1.8199, 18.1117) -> (1.8465, 18.0438)
  line L1743 (1.8465, 18.0438) -> (1.8765, 17.985)
  line L1744 (1.8765, 17.985) -> (1.9096, 17.9354)
  line L1745 (1.9096, 17.9354) -> (1.9454, 17.8951)
  line L1746 (1.9454, 17.8951) -> (1.9836, 17.8643)
  line L1747 (1.9836, 17.8643) -> (2.0238, 17.8429)
  line L1748 (2.0238, 17.8429) -> (2.0761, 17.8295)
  line L1749 (2.0761, 17.8295) -> (2.3902, 17.7902)
  line L1750 (2.3902, 17.7902) -> (2.808, 17.729)
  line L1751 (2.808, 17.729) -> (3.2242, 17.6581)
  line L1752 (3.2242, 17.6581) -> (3.5351, 17.5985)
  line L1753 (3.5351, 17.5985) -> (3.589, 17.5949)
  line L1754 (3.589, 17.5949) -> (3.6338, 17.6029)
  line L1755 (3.6338, 17.6029) -> (3.6797, 17.6205)
  line L1756 (3.6797, 17.6205) -> (3.7262, 17.6477)
  line L1757 (3.7262, 17.6477) -> (3.773, 17.6846)
  line L1758 (3.773, 17.6846) -> (3.8197, 17.7313)
  line L1759 (3.8197, 17.7313) -> (3.866, 17.7876)
  line L1760 (3.866, 17.7876) -> (3.9113, 17.8537)
  line L1761 (3.9113, 17.8537) -> (3.9979, 18.015)
  line L1762 (3.9979, 18.015) -> (4.0764, 18.2149)
  line L1763 (4.0764, 18.2149) -> (4.1257, 18.3792)
  line L1764 (4.1257, 18.3792) -> (4.1835, 18.5448)
  line L1765 (4.1835, 18.5448) -> (4.307, 18.8229)
  line L1766 (4.307, 18.8229) -> (4.3995, 19.0014)
  line L1767 (4.3995, 19.0014) -> (4.5169, 19.2065)
  line L1768 (4.5169, 19.2065) -> (4.6593, 19.4329)
  line L1769 (4.6593, 19.4329) -> (4.8302, 19.6809)
  line L1770 (4.8302, 19.6809) -> (5.0311, 19.9477)
  line L1771 (5.0311, 19.9477) -> (5.263, 20.2304)
  line L1772 (5.263, 20.2304) -> (5.5298, 20.5291)
  line L1773 (5.5298, 20.5291) -> (5.8308, 20.839)
  line L1774 (5.8308, 20.839) -> (6.1345, 21.1274)
  arc A38 (7.4555, 20.6982) -> (6.1345, 21.1274) centre (0, 0) ccw
  line L1775 (7.4555, 20.6982) -> (7.5317, 20.2864)
  line L1776 (7.5317, 20.2864) -> (7.593, 19.8587)
  line L1777 (7.593, 19.8587) -> (7.6332, 19.4602)
  line L1778 (7.6332, 19.4602) -> (7.6547, 19.0953)
  line L1779 (7.6547, 19.0953) -> (7.6604, 18.7613)
  line L1780 (7.6604, 18.7613) -> (7.6529, 18.4602)
  line L1781 (7.6529, 18.4602) -> (7.6351, 18.1934)
  line L1782 (7.6351, 18.1934) -> (7.6095, 17.9584)
  line L1783 (7.6095, 17.9584) -> (7.5794, 17.7596)
  line L1784 (7.5794, 17.7596) -> (7.5158, 17.462)
  line L1785 (7.5158, 17.462) -> (7.4653, 17.2942)
  line L1786 (7.4653, 17.2942) -> (7.4085, 17.1322)
  line L1787 (7.4085, 17.1322) -> (7.3546, 16.9244)
  line L1788 (7.3546, 16.9244) -> (7.3298, 16.743)
  line L1789 (7.3298, 16.743) -> (7.3277, 16.6629)
  line L1790 (7.3277, 16.6629) -> (7.3319, 16.5901)
  line L1791 (7.3319, 16.5901) -> (7.3423, 16.5249)
  line L1792 (7.3423, 16.5249) -> (7.3585, 16.4675)
  line L1793 (7.3585, 16.4675) -> (7.3801, 16.4181)
  line L1794 (7.3801, 16.4181) -> (7.4069, 16.3769)
  line L1795 (7.4069, 16.3769) -> (7.4385, 16.3442)
  line L1796 (7.4385, 16.3442) -> (7.4841, 16.3153)
  line L1797 (7.4841, 16.3153) -> (7.7707, 16.1809)
  line L1798 (7.7707, 16.1809) -> (8.1491, 15.9936)
  line L1799 (8.1491, 15.9936) -> (8.5231, 15.7975)
  line L1800 (8.5231, 15.7975) -> (8.8003, 15.6447)
  line L1801 (8.8003, 15.6447) -> (8.8505, 15.6247)
  line L1802 (8.8505, 15.6247) -> (8.8956, 15.6184)
  line L1803 (8.8956, 15.6184) -> (8.9446, 15.621)